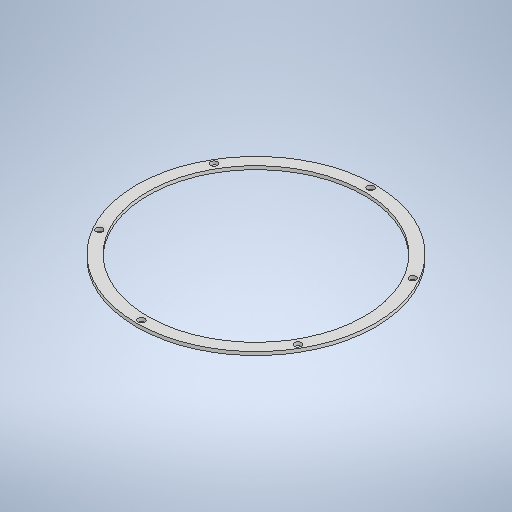
# Autodesk Inventor part: bead lock
Saved by Autodesk Inventor 2025.3 (Build 293356000, 356)
## iProperties
Created: 2026-04-02
Part Number: bead lock
Material: Generic
Document SubType Name: Modeling
Designer: ksawe
Density: 1 g/cm^3
Appearance: Default
Author: ksawe
Autodesk Inventor part; units mm, degrees
ref_plane "YZ Plane" through (0, 0, 0) normal (1, 0, 0) x (0, 1, 0)
ref_plane "XZ Plane" through (0, 0, 0) normal (0, 1, 0) x (-1, 0, 0)
ref_plane "XY Plane" through (0, 0, 0) normal (0, 0, 1) x (1, 0, 0)
sketch "Sketch1" plane through (0, 0, 0) normal (0, 0, 1) x (1, 0, 0)
  circle A0 centre (0, 0) radius 47.5
  circle A1 centre (0, 0) radius 52.5
  circle A2 centre (0, 50.35) radius 1.5
  circle A3 centre (-43.6044, 25.175) radius 1.5
  circle A4 centre (-43.6044, -25.175) radius 1.5
  circle A5 centre (0, -50.35) radius 1.5
  circle A6 centre (43.6044, -25.175) radius 1.5
  circle A7 centre (43.6044, 25.175) radius 1.5
  dimension "d0" = 95
  dimension "d1" = 105
  dimension "d2" = 3
  dimension "d5" = 360
  dimension "d9" = 1.35
  constraints: 8 centre point, 2 coincident, 13 other
  measures "d0" diameter of A0
  measures "d1" diameter of A1
  measures "d2" diameter of A2
extrude "Extrusion1" add sketch "Sketch1" along normal blind 1.5
body "Solid1"
